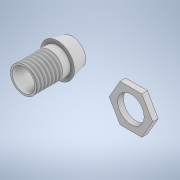
# Autodesk Inventor part: Винтики шпунтики(2 детали)
Saved by Autodesk Inventor 2022 (Build 260153000, 153)
## iProperties
Created: 2022-07-10
Part Number: Винтики шпунтики(2 детали)
Material: Типовые
Document SubType Name: Modeling
Designer: Константин
Density: 1 g/cm^3
Appearance: По умолчанию
Author: Константин
Autodesk Inventor part; units mm, degrees
ref_plane "YZ Plane" through (0, 0, 0) normal (1, 0, 0) x (0, 1, 0)
ref_plane "XZ Plane" through (0, 0, 0) normal (0, 1, 0) x (-1, 0, 0)
ref_plane "XY Plane" through (0, 0, 0) normal (0, 0, 1) x (1, 0, 0)
sketch "Эскиз1" plane through (0, 0, 0) normal (0, 0, 1) x (1, 0, 0)
  circle A0 centre (0, 0) radius 3
  circle A1 centre (0, 0) radius 3.5
  dimension "d0" = 6
  dimension "d1" = 7
  constraints: 2 centre point, 2 coincident
  measures "d0" diameter of A0
  measures "d1" diameter of A1
extrude "Выдавливание1" add sketch "Эскиз1" along normal blind 9
sketch "Эскиз2" plane through (0, 0, 0) normal (0, 0, -1) x (-1, 0, 0)
  circle A0 centre (0, 0) radius 4.5
  dimension "d4" = 9
  constraints: 1 centre point, 1 coincident
  measures "d4" diameter of A0
sketch "Эскиз3" plane through (0, 0, 0) normal (1, 0, 0) x (0, 1, 0)
  line L0 (0, 0) -> (0, -4)
  line L1 (0, -4) -> (3.5, -4)
  line L2 (0, 0) -> (4.5, 0)
  line L3 (3.5, 0) -> (-3.5, 0) projected
  line L4 (4.5, 0) -> (3.5, -4)
  dimension "d5" = 4
  dimension "d6" = 3.5
  dimension "d7" = 4.5
  constraints: 8 end point, 1 collinear, 1 perpendicular, 1 vertical
  measures "d5" distance of L0.start L0.end
  measures "d6" distance of L0.end L1.end
  measures "d7" distance of L0.start L2.end
revolve "Вращение1" add sketch "Эскиз3" angle 360 about axis through (0, 0, 0) along (0, 0, -1)
sketch "Эскиз4" plane through (0, 0, -4) normal (0, 0, -1) x (-1, 0, 0)
  circle A0 centre (0, 0) radius 3.5
  constraints: 1 centre point, 1 coincident
extrude "Выдавливание2" cut sketch "Эскиз4" against normal up to surface (4 mm away)
thread "Резьба1" size "M7x1" class "6g" standard "ANSI Metric M Profile" length 7 offset 2
sketch "Эскиз5" plane through (0, 0, 0) normal (0, 0, 1) x (1, 0, 0)
  line L0 (23.9295, 5) -> (26.8162, 0)
  line L1 (26.8162, 0) -> (23.9295, -5)
  line L2 (23.9295, -5) -> (18.1559, -5)
  line L3 (18.1559, -5) -> (15.2692, 0)
  line L4 (15.2692, 0) -> (18.1559, 5)
  line L5 (18.1559, 5) -> (23.9295, 5)
  point P0 (0, 0)
  point P1 (21.0427, 0)
  dimension "d13" = 10
  constraints: 12 end point, 1 horizontal alignment, 13 other
  measures "d13" distance between parallel lines of L2 L5
extrude "Выдавливание3" add sketch "Эскиз5" along normal blind 1.5
sketch "Эскиз6" plane through (0, 0, 0) normal (0, 0, -1) x (-1, 0, 0)
  line L0 (-26.8162, 0) -> (-23.9295, 5) projected
  line L1 (-18.1559, 5) -> (-15.2692, 0) projected
  line L2 (-26.8162, 0) -> (-15.2692, 0)
  circle A0 centre (-21.0427, 0) radius 3.5
  point P0 (0, 0)
  dimension "d16" = 7
  constraints: 2 end point, 1 centre point, 1 horizontal, 1 midpoint
  measures "d16" diameter of A0
extrude "Выдавливание4" cut sketch "Эскиз6" against normal through all
